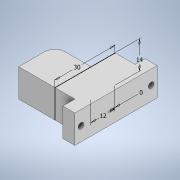
# Autodesk Inventor part: AdaptadorSensorAnycubic
Saved by Autodesk Inventor 2020.3 (Build 243373000, 373)
## iProperties
Created: 2020-09-07
Part Number: AdaptadorSensorAnycubic
Material: Generic
Document SubType Name: Modeling
Designer: mifer
Density: 1 g/cm^3
Appearance: Default
Author: mifer
## iProperties of the stored document _3DPrint.ipt
Created: 2020-09-09
Part Number: _3DPrint
Material: Generic
Document SubType Name: Modeling
Designer: mifer
Density: 1 g/cm^3
Appearance: Default
Author: mifer
Autodesk Inventor part; units mm, degrees
ref_plane "YZ Plane" through (0, 0, 0) normal (1, 0, 0) x (0, 1, 0)
ref_plane "XZ Plane" through (0, 0, 0) normal (0, 1, 0) x (-1, 0, 0)
ref_plane "XY Plane" through (0, 0, 0) normal (0, 0, 1) x (1, 0, 0)
sketch "Sketch1" plane through (0, 0, 0) normal (1, 0, 0) x (0, 1, 0)
  line L0 (0, 0) -> (14, 0)
  line L1 (14, 0) -> (14, -30)
  line L2 (14, -30) -> (0, -30)
  line L3 (0, -30) -> (0, 0)
  line L4 (14, -30) -> (0, -30)
  line L5 (0, -30) -> (0, -30)
  line L6 (0, -30) -> (14, -30)
  line L7 (14, -30) -> (14, -30)
  line L8 (0, 0) -> (0, -18)
  line L9 (0, -18) -> (14, -18)
  line L10 (14, -18) -> (14, 0)
  point P0 (14, -18)
  dimension "d12" = 14
  dimension "d13" = 30
  dimension "d14" = 12
  dimension "d15" = 0
  constraints: 22 end point, 5 equal length, 3 point on line, 2 horizontal, 2 perpendicular
  measures "d12" distance of L1.end L2.end
  measures "d13" distance of L0.end L1.end
  measures "d14" distance between parallel lines of L4 L9
  measures "d15" distance between parallel lines of L2 L4
extrude "Extrusion6" add sketch "Sketch1" along normal blind 10 contours L9 L1 L2 L3
extrude "Extrusion7" add sketch "Sketch1" along normal blind 10 and the other way blind 18 contours L0 L1 L9 L3
fillet "Fillet2" radius 5 1 edges at (-18, 7, -18)
sketch "Sketch7" plane through (10, 0, 0) normal (1, 0, 0) x (0, 0, -1)
  line L0 (35, 14) -> (-6, 14)
  line L1 (-6, 14) -> (-6, 0)
  line L2 (-6, 0) -> (35, 0)
  line L3 (35, 0) -> (35, 14)
  line L4 (30, 0) -> (30, 14) projected
  circle A0 centre (32, 7) radius 1.4
  circle A1 centre (-3, 7) radius 1.4
  point P0 (0, 0)
  dimension "d32" = 41
  dimension "d33" = 5
  dimension "d34" = 14
  dimension "d35" = 2.8
  dimension "d36" = 3
  dimension "d37" = 2.8
  dimension "d38" = 35
  constraints: 8 end point, 2 centre point, 2 parallel, 1 horizontal, 1 perpendicular
  measures "d32" distance between parallel lines of L3 L1
  measures "d33" distance between parallel lines of L3 L4
  measures "d34" distance between parallel lines of L2 L0
  measures "d35" diameter of A0
  measures "d36" distance from line of L3 A0.centre
  measures "d37" diameter of A1
  measures "d38" distance of A0.centre A1.centre
extrude "Extrusion9" add sketch "Sketch7" along normal blind 6
body "Solid2"
